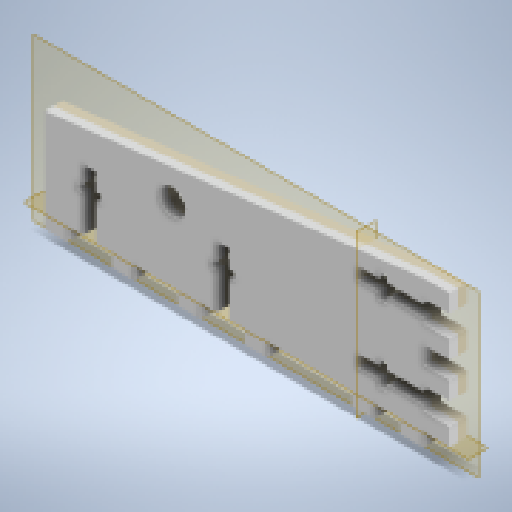
# Autodesk Inventor part: Ребро жётскости крыла
Saved by Autodesk Inventor 2023.2 (Build 272271030, 271C)
## iProperties
Created: 2024-03-20
Part Number: Ребро жётскости крыла
Material: Типовые
Document SubType Name: Modeling
Designer: I9232
Density: 1 g/cm^3
Appearance: По умолчанию
Author: I9232
Autodesk Inventor part; units mm, degrees
sketch "Эскиз1" plane through (0, 0, 0) normal (0, 0, 1) x (1, 0, 0)
  line L0 (-70.2411, 0) -> (14.7589, 0)
  line L1 (14.7589, 0) -> (14.7589, 30)
  line L2 (14.7589, 30) -> (-70.2411, 20)
  line L3 (0, 36) -> (0, -6) construction
  line L4 (-70.2411, 20) -> (-70.2411, 0)
  point P0 (0, 0)
  dimension "d0" = 30
  dimension "d1" = 85
  dimension "d46" = 14.7589
  dimension "d47" = 20
  constraints: 8 end point, 2 horizontal, 1 perpendicular, 1 vertical
  measures "d0" distance of L0.end L1.end
  measures "d1" distance of L0.start L0.end
  measures "d46" distance between parallel lines of L1 L3
  measures "d47" distance of L2.end L0.start
extrude "Выдавливание1" add sketch "Эскиз1" along normal mid plane 4
sketch "Эскиз2" plane through (-70.2411, 0, 2) normal (0, -1, 0) x (1, 0, 0)
  line L0 (0, -4) -> (0, 0) projected
  line L1 (85, 0) -> (0, 0) projected
  line L2 (0, -4) -> (5, -4)
  line L3 (5, -4) -> (5, 0)
  line L4 (5, 0) -> (0, 0)
  line L5 (0, 0) -> (0, -4)
  line L6 (0, -4) -> (85, -4) projected
  line L7 (15, -4) -> (20, -4)
  line L8 (20, -4) -> (20, 0)
  line L9 (20, 0) -> (15, 0)
  line L10 (15, 0) -> (15, -4)
  line L11 (30, -4) -> (35, -4)
  line L12 (35, -4) -> (35, 0)
  line L13 (35, 0) -> (30, 0)
  line L14 (30, 0) -> (30, -4)
  line L15 (45, -4) -> (50, -4)
  line L16 (50, -4) -> (50, 0)
  line L17 (50, 0) -> (45, 0)
  line L18 (45, 0) -> (45, -4)
  line L19 (85, -4) -> (80, -4)
  line L20 (80, -4) -> (80, 0)
  line L21 (80, 0) -> (85, 0)
  line L22 (85, 0) -> (85, -4)
  line L23 (74, -4) -> (69, -4)
  line L24 (69, -4) -> (69, 0)
  line L25 (69, 0) -> (74, 0)
  line L26 (74, 0) -> (74, -4)
  point P0 (70.2411, -2)
  point P1 (15, 0)
  point P2 (45, 0)
  point P3 (74, 0)
  dimension "d4" = 5
  dimension "d5" = 5
  dimension "d6" = 10
  dimension "d9" = 30
  dimension "d14" = 5
  dimension "d15" = 5
  dimension "d16" = 6
  constraints: 48 end point, 8 parallel, 6 point on line, 5 horizontal, 4 perpendicular, 16 other
  measures "d4" distance of L0.start L2.end
  measures "d5" distance of L7.start L7.end
  measures "d6" distance between parallel lines of L3 L10
  measures "d9" distance of L3.end L12.end
  measures "d14" distance of L19.end L6.end
  measures "d15" distance of L23.end L23.start
  measures "d16" distance between parallel lines of L26 L20
extrude "Выдавливание2" add sketch "Эскиз2" along normal blind 3 contours L0 L1 L3 L2 | L10 L1 L8 L6 | L14 L1 L12 L6 | L18 L1 L16 L6 | L24 L1 L26 L6 | L20 L1 L22 L6
sketch "Эскиз3" plane through (14.7589, 30, 2) normal (1, 0, 0) x (0, 0, -1)
  line L0 (4, 0) -> (0, 0) projected
  line L1 (4, 0) -> (0, 0)
  line L2 (0, 0) -> (0, -4)
  line L3 (0, -4) -> (4, -4)
  line L4 (4, -4) -> (4, 0)
  line L5 (4, -9) -> (0, -9)
  line L6 (0, -9) -> (0, -13)
  line L7 (0, -13) -> (4, -13)
  line L8 (4, -13) -> (4, -9)
  line L9 (4, 0) -> (4, -33) projected
  line L10 (4, -10) -> (4, 0) projected
  line L11 (0, 0) -> (0, -33) projected
  line L12 (4, -17) -> (0, -17)
  line L13 (0, -17) -> (0, -21)
  line L14 (0, -21) -> (4, -21)
  line L15 (4, -21) -> (4, -17)
  line L16 (4, -26) -> (0, -26)
  line L17 (0, -26) -> (0, -30)
  line L18 (0, -30) -> (4, -30)
  line L19 (4, -30) -> (4, -26)
  point P0 (2, -30)
  point P1 (4, -30)
  point P2 (4, -16.5)
  point P3 (4, -30)
  point P4 (0, -26)
  point P5 (0, -17)
  dimension "d19" = 4
  dimension "d20" = 4
  dimension "d21" = 5
  dimension "d29" = 4
  dimension "d30" = 5
  dimension "d31" = 4
  dimension "d32" = 4
  constraints: 32 end point, 8 parallel, 4 horizontal, 4 perpendicular, 4 point on line, 3 other
  measures "d19" distance of L3.end L0.start
  measures "d20" distance of L7.end L5.start
  measures "d21" distance between parallel lines of L5 L3
  measures "d29" distance of L18.end L16.start
  measures "d30" distance between parallel lines of L16 L14
  measures "d31" distance between parallel lines of L12 L7
  measures "d32" distance of L14.end L12.start
extrude "Выдавливание3" add sketch "Эскиз3" along normal blind 6 contours L4 L3 L2 L0 | L8 L7 L6 L5 | L12 L9 L14 L11 | L16 L9 L18 L11
sketch "Эскиз4" plane through (0, 0, 2) normal (0, 0, 1) x (1, 0, 0)
  line L0 (-0.1411, 5.05) -> (-0.1411, 7.95)
  line L1 (14.7589, 7.95) -> (14.7589, 5.05)
  line L2 (6.6589, 9.3) -> (4.8589, 9.3)
  line L3 (4.8589, 3.7) -> (6.6589, 3.7)
  line L4 (14.7589, 9) -> (14.7589, 4) projected
  line L5 (14.7589, 6.5) -> (-0.1411, 6.5) construction
  line L6 (-0.1411, 7.95) -> (4.8589, 7.95)
  line L7 (6.6589, 7.95) -> (14.7589, 7.95)
  line L8 (6.6589, 3.7) -> (6.6589, 5.05)
  line L9 (6.6589, 7.95) -> (6.6589, 9.3)
  line L10 (4.8589, 9.3) -> (4.8589, 7.95)
  line L11 (4.8589, 5.05) -> (4.8589, 3.7)
  line L12 (14.7589, 5.05) -> (6.6589, 5.05)
  line L13 (4.8589, 5.05) -> (-0.1411, 5.05)
  line L14 (-0.1411, 22.05) -> (-0.1411, 24.95)
  line L15 (14.7589, 24.95) -> (14.7589, 22.05)
  line L16 (6.6589, 26.3) -> (4.8589, 26.3)
  line L17 (4.8589, 20.7) -> (6.6589, 20.7)
  line L18 (14.7589, 23.5) -> (-0.1411, 23.5) construction
  line L19 (-0.1411, 24.95) -> (4.8589, 24.95)
  line L20 (6.6589, 24.95) -> (14.7589, 24.95)
  line L21 (6.6589, 20.7) -> (6.6589, 22.05)
  line L22 (6.6589, 24.95) -> (6.6589, 26.3)
  line L23 (4.8589, 26.3) -> (4.8589, 24.95)
  line L24 (4.8589, 22.05) -> (4.8589, 20.7)
  line L25 (14.7589, 22.05) -> (6.6589, 22.05)
  line L26 (4.8589, 22.05) -> (-0.1411, 22.05)
  line L27 (14.7589, 26) -> (14.7589, 21) projected
  point P0 (0, 0)
  dimension "d33" = 2.9
  dimension "d34" = 1.8
  dimension "d35" = 5.6
  dimension "d37" = 1.35
  dimension "d38" = 5
  dimension "d39" = 8.1
  dimension "d40" = 2.9
  dimension "d41" = 1.8
  dimension "d42" = 5.6
  dimension "d43" = 1.35
  dimension "d44" = 5
  dimension "d45" = 8.1
  constraints: 52 end point, 20 parallel, 8 equal length, 8 midpoint, 8 perpendicular, 6 horizontal, 1 coincident
  measures "d33" distance of L0.start L0.end
  measures "d34" distance of L3.start L3.end
  measures "d35" distance of L3.end L2.start
  measures "d37" distance of L11.start L3.start
  measures "d38" distance of L0.end L6.end
  measures "d39" distance of L7.start L1.start
  measures "d40" distance of L14.start L19.start
  measures "d41" distance of L17.start L21.start
  measures "d42" distance of L21.start L22.end
  measures "d43" distance of L24.start L17.start
  measures "d44" distance of L19.start L19.end
  measures "d45" distance of L22.start L15.start
extrude "Выдавливание4" cut sketch "Эскиз4" against normal up to surface (4 mm away)
sketch "Эскиз5" plane through (0, 0, 2) normal (0, 0, 1) x (1, 0, 0)
  line L0 (-61.6911, 0) -> (-58.7911, 0)
  line L1 (-58.7911, 13.9) -> (-61.6911, 13.9)
  line L2 (-31.6911, 0) -> (-28.7911, 0)
  line L3 (-28.7911, 13.9) -> (-31.6911, 13.9)
  line L4 (-60.2411, 0) -> (-60.2411, 13.9) construction
  line L5 (-30.2411, 13.9) -> (-30.2411, 0) construction
  line L6 (-57.4411, 9.9) -> (-57.4411, 8.1)
  line L7 (-63.0411, 8.1) -> (-63.0411, 9.9)
  line L8 (-27.4411, 9.9) -> (-27.4411, 8.1)
  line L9 (-33.0411, 8.1) -> (-33.0411, 9.9)
  line L10 (-63.0411, 9.9) -> (-61.6911, 9.9)
  line L11 (-58.7911, 9.9) -> (-57.4411, 9.9)
  line L12 (-61.6911, 13.9) -> (-61.6911, 9.9)
  line L13 (-61.6911, 8.1) -> (-61.6911, 0)
  line L14 (-57.4411, 8.1) -> (-58.7911, 8.1)
  line L15 (-61.6911, 8.1) -> (-63.0411, 8.1)
  line L16 (-58.7911, 0) -> (-58.7911, 8.1)
  line L17 (-58.7911, 9.9) -> (-58.7911, 13.9)
  line L18 (-33.0411, 9.9) -> (-31.6911, 9.9)
  line L19 (-28.7911, 9.9) -> (-27.4411, 9.9)
  line L20 (-27.4411, 8.1) -> (-28.7911, 8.1)
  line L21 (-31.6911, 8.1) -> (-33.0411, 8.1)
  line L22 (-31.6911, 13.9) -> (-31.6911, 9.9)
  line L23 (-31.6911, 8.1) -> (-31.6911, 0)
  line L24 (-28.7911, 0) -> (-28.7911, 8.1)
  line L25 (-28.7911, 9.9) -> (-28.7911, 13.9)
  line L26 (-65.2411, 0) -> (-55.2411, 0) projected
  line L27 (-35.2411, 0) -> (-25.2411, 0) projected
  point P0 (0, 0)
  dimension "d50" = 1.8
  dimension "d51" = 5.6
  dimension "d52" = 2.9
  dimension "d54" = 1.35
  dimension "d55" = 8.1
  dimension "d56" = 4
  constraints: 52 end point, 20 parallel, 14 equal length, 8 perpendicular, 6 horizontal, 6 midpoint
  measures "d50" distance of L6.start L6.end
  measures "d51" distance of L7.end L6.start
  measures "d52" distance of L1.start L1.end
  measures "d54" distance of L11.start L6.start
  measures "d55" distance of L0.end L14.end
  measures "d56" distance of L1.end L10.end
extrude "Выдавливание5" cut sketch "Эскиз5" against normal up to surface (4 mm away)
sketch "Эскиз6" plane through (0, 0, -2) normal (0, 0, -1) x (-1, 0, 0)
  circle A0 centre (41.6053, 16.5) radius 2
  point P0 (0, 0)
  dimension "d61" = 4
  constraints: 1 centre point, 1 other
  measures "d61" diameter of A0
extrude "Выдавливание6" cut sketch "Эскиз6" against normal up to surface (4 mm away)
